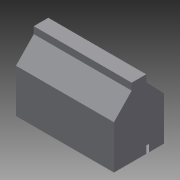
# Autodesk Inventor part: BE 2
Saved by Autodesk Inventor 2013 (Build 170138000, 138)
## iProperties
Created: 2006-05-01
Part Number: BE 2
Document SubType Name: Modeling
Designer: mcgratta
Material: Generic
Density: 1 g/cm^3
Author: mcgratta
Autodesk Inventor part; units mm, degrees
ref_plane "YZ Plane" through (0, 0, 0) normal (1, 0, 0) x (0, 1, 0)
ref_plane "XZ Plane" through (0, 0, 0) normal (0, 1, 0) x (-1, 0, 0)
ref_plane "XY Plane" through (0, 0, 0) normal (0, 0, 1) x (1, 0, 0)
sketch "Sketch1" plane through (0, 0, 0) normal (0, 0, 1) x (1, 0, 0)
  line L0 (0, 13800) -> (27000, 13800)
  line L1 (27000, 13800) -> (27000, 0)
  line L2 (27000, 0) -> (0, 0)
  line L3 (0, 0) -> (0, 13800)
  dimension "d0" = 13800
  dimension "d1" = 27000
  constraints: 8 end point, 2 parallel, 1 horizontal, 1 perpendicular
  measures "d0" distance of L2.end L0.start
  measures "d1" distance of L0.start L0.end
extrude "Extrusion1" add sketch "Sketch1" along normal blind 19000
sketch "Sketch2" plane through (27000, 0, 0) normal (1, 0, 0) x (0, 0, -1)
  line L0 (-19000, 13800) -> (-19000, 0) projected
  line L1 (0, 0) -> (-19000, 0) projected
  line L2 (0, 13800) -> (0, 0) projected
  line L3 (0, 13800) -> (-19000, 13800) projected
  line L4 (-4000, 9700) -> (0, 9700)
  line L5 (0, 9700) -> (0, 8900)
  line L6 (0, 8900) -> (-4000, 8900)
  line L7 (-4000, 8900) -> (-4000, 9700)
  line L8 (-19000, 8900) -> (-17100, 8900)
  line L9 (-17100, 8900) -> (-12000, 13800)
  line L10 (-19000, 4900) -> (-17100, 4900)
  line L11 (-17100, 4900) -> (-12000, 0)
  dimension "d4" = 4000
  dimension "d5" = 800
  dimension "d6" = 8900
  dimension "d7" = 4900
  dimension "d9" = 12000
  dimension "d11" = 1900
  dimension "d13" = 1900
  dimension "d14" = 4900
  dimension "d15" = 12000
  constraints: 16 end point, 5 point on line, 3 parallel, 2 perpendicular, 1 horizontal
  measures "d4" distance of L4.start L4.end
  measures "d5" distance of L6.end L4.start
  measures "d6" distance between parallel lines of L1 L6
  measures "d7" distance between parallel lines of L3 L8
  measures "d9" distance from line of L2 L9.end
  measures "d11" distance of L8.start L8.end
  measures "d13" distance of L10.start L10.end
  measures "d14" distance between parallel lines of L1 L10
  measures "d15" distance from line of L2 L11.end
extrude "Extrusion2" cut sketch "Sketch2" against normal through all contours L3 L9 L8 L0
extrude "Extrusion3" cut sketch "Sketch2" against normal through all contours L10 L11 L1 L0
sketch "Sketch3" plane through (0, 0, 0) normal (-1, 0, 0) x (0, 0, 1)
  line L0 (0, 0) -> (0, 13800) projected
  line L1 (0, 0) -> (12000, 0) projected
  line L2 (0, 9700) -> (4000, 9700)
  line L3 (4000, 9700) -> (4000, 8900)
  line L4 (4000, 8900) -> (0, 8900)
  line L5 (0, 8900) -> (0, 9700)
  dimension "d20" = 4000
  dimension "d21" = 800
  dimension "d22" = 8900
  constraints: 8 end point, 2 parallel, 1 horizontal, 1 perpendicular, 1 point on line
  measures "d20" distance of L3.end L4.end
  measures "d21" distance of L2.end L3.end
  measures "d22" distance between parallel lines of L1 L4
shell "Shell1" thickness 1 removed faces 0
extrude "Extrusion4" cut sketch "Sketch2" against normal mid plane 3 contours L2 L6 L7 L4
extrude "Extrusion5" cut sketch "Sketch3" against normal mid plane 3
sketch "Sketch4" plane through (0, 0, 0) normal (0, 0, -1) x (-1, 0, 0)
  line L0 (0, 9700) -> (0, 13800) projected
  line L1 (-27000, 0) -> (0, 0) projected
  line L2 (0, 0) -> (0, 8900) projected
  line L3 (-25000, 12500) -> (-18000, 12500)
  line L4 (-18000, 12500) -> (-18000, 9700)
  line L5 (-18000, 9700) -> (-25000, 9700)
  line L6 (-25000, 9700) -> (-25000, 12500)
  line L7 (-6200, 12500) -> (-1200, 12500)
  line L8 (-1200, 12500) -> (-1200, 9700)
  line L9 (-1200, 9700) -> (-6200, 9700)
  line L10 (-6200, 9700) -> (-6200, 12500)
  circle A0 centre (-16000, 7200) radius 600
  circle A1 centre (-16000, 7200) radius 800
  dimension "d28" = 2800
  dimension "d29" = 7000
  dimension "d30" = 18000
  dimension "d31" = 9700
  dimension "d32" = 5000
  dimension "d33" = 2800
  dimension "d34" = 1200
  dimension "d35" = 9700
  dimension "d36" = 1200
  dimension "d37" = 7200
  dimension "d38" = 16000
  dimension "d39" = 1600
  constraints: 16 end point, 4 parallel, 2 centre point, 2 horizontal, 2 perpendicular, 1 coincident
  measures "d28" distance of L5.end L3.start
  measures "d29" distance of L4.end L5.end
  measures "d30" distance between parallel lines of L0 L4
  measures "d31" distance between parallel lines of L1 L5
  measures "d32" distance of L8.end L9.end
  measures "d33" distance of L9.end L7.start
  measures "d34" distance between parallel lines of L0 L8
  measures "d35" distance between parallel lines of L1 L9
  measures "d36" diameter of A0
  measures "d37" distance from line of L1 A0.centre
  measures "d38" distance from line of L2 A0.centre
  measures "d39" diameter of A1
extrude "Extrusion6" add sketch "Sketch4" against normal blind 9400 contours L7 L8 L9 L10
extrude "Extrusion7" add sketch "Sketch4" against normal blind 4000 contours L3 L4 L5 L6
extrude "Extrusion8" add sketch "Sketch4" against normal blind 1000 contours A1
body "Solid1"
